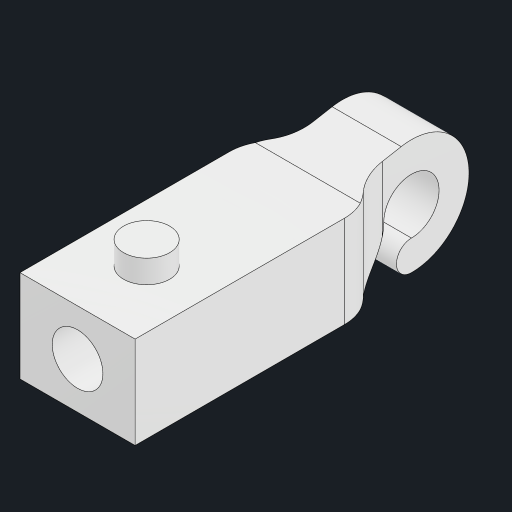
# Autodesk Inventor part: gear_connecotr1_V2
Saved by Autodesk Inventor 2023 (Build 270158000, 158)
## iProperties
Created: 2022-06-15
Part Number: gear_connecotr1_V2
Material: ABS プラスチック
Document SubType Name: Modeling
Designer: legot
Density: 1.06 g/cm^3
Appearance: 滑らか - 白
Mass: 0.227309 g
Surface Area: 3.88253 cm^2
Volume: 0.214443 cm^3
Author: legot
Autodesk Inventor part; units mm, degrees
ref_plane "YZ Plane" through (0, 0, 0) normal (1, 0, 0) x (0, 1, 0)
ref_plane "XZ Plane" through (0, 0, 0) normal (0, 1, 0) x (-1, 0, 0)
ref_plane "XY Plane" through (0, 0, 0) normal (0, 0, 1) x (1, 0, 0)
sketch "スケッチ1" plane through (0, 0, 0) normal (0, 1, 0) x (-1, 0, 0)
  line L0 (2.5, 3) -> (-2.5, 3)
  line L1 (-2.5, 3) -> (-2.5, -7)
  line L2 (-2.5, -7) -> (2.5, -7)
  line L3 (2.5, -7) -> (2.5, 3)
  point P0 (0, 0)
  point P1 (0, 3)
  dimension "d0" = 5
  dimension "d15" = 10
  dimension "d46" = 3
  constraints: 8 end point, 2 parallel, 1 horizontal, 1 midpoint, 1 perpendicular, 1 vertical alignment
  measures "d0" distance of L0.start L0.end
  measures "d15" distance of L2.end L0.start
  measures "d46" distance from line of point (0, 0) L0
extrude "押し出し1" add sketch "スケッチ1" along normal mid plane 4
sketch "スケッチ2" plane through (0, 0, 0) normal (0, 1, 0) x (-1, 0, 0)
  circle A0 centre (0, 0) radius 1
  dimension "d3" = 2
  constraints: 1 centre point, 1 coincident
  measures "d3" diameter of A0
extrude "押し出し2" add sketch "スケッチ2" along normal mid plane 6
sketch "スケッチ5" plane through (-2.5, 2, 3) normal (0, 0, 1) x (1, 0, 0)
  point P0 (2.5, -2)
  point P1 (2.5, -2)
  constraints: 1 coincident
hole "加工用" [suppressed]
sketch "スケッチ8" plane through (0, 0, 0) normal (1, 0, 0) x (0, 1, 0)
  circle A0 centre (0, -10) radius 2.5
  circle A1 centre (0, -10) radius 1.2
  line L0 (-2, -7) -> (-2.4604, -9.557)
  line L1 (2, -7) -> (2.4604, -9.557)
  line L2 (-2, -7) -> (2, -7) projected
  line L3 (-2, -7) -> (2, -7) projected
  circle A2 centre (-1.85, -10) radius 0.65
  arc A3 (-2, -7) -> (0, -8.8) centre (0, -6.7889) ccw
  point P0 (0, 0)
  point P1 (1, -4)
  point P2 (-1, -4)
  point P3 (0, -7)
  point P4 (0, -7)
  point P5 (-1.2, -10)
  point P6 (-2.5, -10)
  point P7 (0, -7)
  point P8 (-1.5657, -8.051)
  dimension "d33" = 2.4
  dimension "d34" = 5
  dimension "d42" = 3
  constraints: 4 end point, 4 point on circle, 3 centre point, 3 coincident, 3 tangent, 2 vertical alignment, 1 horizontal alignment, 10 other
  measures "d34" diameter of A0
  measures "d42" distance of A0.centre point (0, -7)
extrude "押し出し4" add sketch "スケッチ8" along normal mid plane 3 contours A0 A2 A1 A3 | A0 A3 L2 L1 | A2 picked at (-1.463, -11.0204)
fillet "フィレット1" radius 2 4 edges at (-1.5, 0, -7) (-2.5, 0, -7) (1.5, 0, -7) (2.5, 0, -7)
sketch "スケッチ6" plane through (-2.5, 2, 3) normal (0, 0, 1) x (1, 0, 0)
  point P0 (2.5, -2)
  point P1 (2.5, -2)
  constraints: 1 coincident
hole "穴3" at (0, 0, 3) direction (0, 0, -1) diameter 2.2 end up to face face through (0, 0, -10) facing (1, 0, 0) round with radius 1.2 far side no
